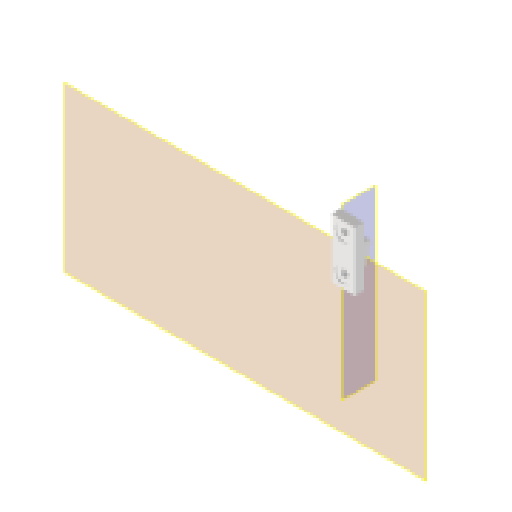
# Autodesk Inventor part: Holisheet_tubeclamp
Saved by Autodesk Inventor 2025.3 (Build 293356000, 356)
## iProperties
Created: 2023-03-24
Part Number: Holisheet_tubeclamp
Material: Generisch
Document SubType Name: Modeling
Designer: diederichbenedict
Density: 1 g/cm^3
Appearance: Vorgabe
Author: diederichbenedict
Autodesk Inventor part; units mm, degrees
ref_plane "YZ Plane" through (0, 0, 0) normal (1, 0, 0) x (0, 1, 0)
ref_plane "XZ Plane" through (0, 0, 0) normal (0, 1, 0) x (-1, 0, 0)
ref_plane "XY Plane" through (0, 0, 0) normal (0, 0, 1) x (1, 0, 0)
ref_plane "Arbeitsebene1" through (0, 0, 0) normal (0, 0, 1) x (1, 0, 0)
ref_plane "Arbeitsebene2" through (37.9, 18.5, 0) normal (-1, 0, 0) x (0, -1, 0)
sketch "Skizze1" plane through (37.9, 18.5, 0) normal (-1, 0, 0) x (0, -1, 0)
  line L0 (5.15, -4.875) -> (5.15, 0) projected
  line L1 (13.35, 0) -> (59.85, 0) projected
  line L2 (13.35, 0) -> (13.35, -4.875) projected
  arc A0 (5.15, -4.875) -> (13.35, -4.875) centre (9.25, -4.875) ccw projected
  circle A1 centre (9.25, -4.875) radius 4
  line L3 (5.25, -4.875) -> (13.25, -4.875)
  line L4 (13.25, -4.875) -> (13.25, 1)
  line L5 (13.25, 1) -> (5.25, 1)
  line L6 (5.25, 1) -> (5.25, -4.875)
  line L7 (20.25, 4.5) -> (-1.75, 4.5)
  line L8 (-1.75, 4.5) -> (-1.75, 1)
  line L9 (-1.75, 1) -> (20.25, 1)
  line L10 (20.25, 1) -> (20.25, 4.5)
  line L11 (20.25, 4.5) -> (-1.75, 1) construction
  line L12 (-1.75, 4.5) -> (20.25, 1) construction
  line L13 (20.25, 4.5) -> (21.25, 4.5)
  line L14 (21.25, 4.5) -> (21.25, 1)
  line L15 (21.25, 1) -> (20.25, 1)
  line L16 (20.25, 1) -> (20.25, 4.5)
  line L17 (59.85, -17) -> (-8, -17) projected
  line L18 (59.85, 0) -> (59.85, -17) projected
  line L19 (-8, 0) -> (5.15, 0) projected
  line L20 (-8, -17) -> (-8, 0) projected
  point P0 (18.5, 0)
  point P1 (0, 0)
  point P2 (59.85, -12)
  point P3 (9.25, 2.75)
  point P4 (13.25, -4.875)
  point P5 (13.25, 1)
  dimension "d0" = 8
  dimension "d1" = 1
  dimension "d2" = 3.5
  dimension "d3" = 11
  dimension "d14" = 1
  constraints: 28 end point, 6 parallel, 3 horizontal, 3 perpendicular, 2 midpoint, 1 coincident, 1 point on line, 3 other
  measures "d1" distance from line of L5 L0.end
  measures "d2" distance between parallel lines of L7 L5
  measures "d3" distance from line of L8 point (9.25, 2.75)
  measures "d14" distance of L14.end L15.end
extrude "Extrusion1" add sketch "Skizze1" against normal blind 9 contours A1 L6 L5 L4 | L5 L9 L8 L7 L10 | L10 L13 L14 L15
sketch "Skizze2" plane through (37.9, -1.75, 4.5) normal (0, 0, 1) x (1, 0, 0)
  circle A0 centre (4.5, 18) radius 1.4 projected
  circle A1 centre (4.5, 4) radius 1.4 projected
  point P0 (-37.9, 1.75)
hole "Bohrung1" at (42.4, 16.25, 4.5) at (42.4, 2.25, 4.5) direction (0, 0, -1) diameter 2.8 depth 8 tip angle 118 counterbore diameter 6.5 counterbore depth 0.5
fillet "Rundung1" radius 1 2 edges at (42.4, 13.25, -4.875) (42.4, 5.25, -4.875)
